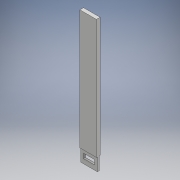
# Autodesk Inventor part: switcher
Saved by Autodesk Inventor 2018 (Build 220112000, 112)
## iProperties
Created: 2017-12-09
Part Number: switcher
Material: Generic
Document SubType Name: Modeling
Designer: ragna
Density: 1 g/cm^3
Appearance: Default
phheight: 6,000 mm
phwidth: 2,500 mm
phtofree: 2,500 mm
phtosolid: 2,000 mm
pheight: 9,000 mm
Author: ragna
Autodesk Inventor part; units mm, degrees
ref_plane "YZ Plane" through (0, 0, 0) normal (1, 0, 0) x (0, 1, 0)
ref_plane "XZ Plane" through (0, 0, 0) normal (0, 1, 0) x (-1, 0, 0)
ref_plane "XY Plane" through (0, 0, 0) normal (0, 0, 1) x (1, 0, 0)
sketch "Sketch8" plane through (0, 0, 0) normal (0, 1, 0) x (-1, 0, 0)
  line L0 (4.5, 0) -> (-4.5, 0)
  line L1 (-4.5, 0) -> (-4.5, -65)
  line L2 (-4.5, -65) -> (4.5, -65)
  line L3 (4.5, -65) -> (4.5, 0)
  point P0 (0, 0)
  point P1 (0, 0)
  dimension "d46" = 65
  dimension "pheight" = 9
  constraints: 8 end point, 2 parallel, 1 coincident, 1 horizontal, 1 midpoint, 1 perpendicular
  measures "d46" distance of L2.end L0.start
  measures "pheight" distance of L0.start L0.end
extrude "Extrusion8" add sketch "Sketch8" along normal blind 2
sketch "Sketch9" plane through (4.5, 0, -65) normal (0, 0, -1) x (-1, 0, 0)
  line L0 (9, 0) -> (9, 2) projected
  line L1 (0, 0) -> (0, 2) projected
  line L2 (9, 1.5) -> (0, 1.5)
  line L3 (0, 1.5) -> (0, 0.5)
  line L4 (0, 0.5) -> (9, 0.5)
  line L5 (9, 0.5) -> (9, 1.5)
  line L6 (0, 2) -> (9, 2) projected
  line L7 (0, 0) -> (9, 0) projected
  point P0 (4.5, 0)
  dimension "d50" = 0.5
  dimension "d51" = 0.5
  dimension "d52" = 1
  constraints: 8 end point, 2 parallel, 2 point on line, 1 horizontal, 1 perpendicular
  measures "d50" distance between parallel lines of L6 L2
  measures "d51" distance between parallel lines of L7 L4
  measures "d52" distance between parallel lines of L2 L4
extrude "Extrusion9" add sketch "Sketch9" along normal blind 7 contours L4 L1 L2 L0
sketch "Sketch10" plane through (-4.5, 1.5, -65) normal (0, 1, 0) x (1, 0, 0)
  line L0 (1.5, 2) -> (7.5, 2)
  line L1 (7.5, 2) -> (7.5, 4.5)
  line L2 (7.5, 4.5) -> (1.5, 4.5)
  line L3 (1.5, 4.5) -> (1.5, 2)
  line L4 (0, 0) -> (0, 7) projected
  line L5 (9, 0) -> (9, 7) projected
  line L6 (0, 7) -> (9, 7) projected
  line L7 (9, 0) -> (0, 0) projected
  point P0 (4.5, -65)
  dimension "d55" = 1.5
  dimension "d56" = 1.5
  dimension "phheight" = 6
  dimension "phwidth" = 2.5
  dimension "phtofree" = 2.5
  dimension "phtosolid" = 2
  constraints: 8 end point, 2 parallel, 1 horizontal, 1 perpendicular
  measures "d55" distance between parallel lines of L4 L3
  measures "d56" distance between parallel lines of L5 L1
  measures "phheight" distance between parallel lines of L1 L3
  measures "phwidth" distance of L2.end L0.start
  measures "phtofree" distance between parallel lines of L6 L2
  measures "phtosolid" distance between parallel lines of L7 L0
extrude "Extrusion10" cut sketch "Sketch10" against normal blind 7 contours L3 L2 L1 L0
equation "\"d51\" = d50"
equation "\"d56\" = d55"
body "Solid2"
